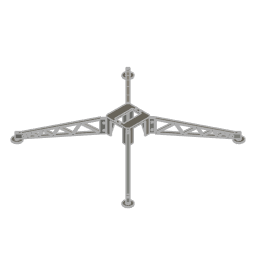
nerfaccelp3 v7 (Autodesk Fusion 360 design; units mm, degrees)
Autodesk Fusion 360 part; units mm, degrees
sketch "Sketch1" plane through (0, 0, 0) normal (0, 0, 1) x (1, 0, 0)
  line L0 (0, 0) -> (54, 0)
  line L1 (54, 0) -> (54, -54)
  line L2 (54, -54) -> (0, -54)
  line L3 (0, -54) -> (0, 0)
  line L4 (16.75, -6.5) -> (37.25, -6.5)
  line L5 (37.25, -6.5) -> (37.25, -47.5)
  line L6 (37.25, -47.5) -> (16.75, -47.5)
  line L7 (16.75, -47.5) -> (16.75, -6.5)
  line L8 (32, -2.725) -> (32, -51.275)
  line L9 (24.15, -2.725) -> (29.85, -2.725)
  line L10 (19.85, -2.725) -> (34.15, -2.725)
  circle A0 centre (32, -2.725) radius 2.15
  line L11 (22, -2.725) -> (32, -51.275)
  line L12 (37.25, -27) -> (16.75, -27)
  circle A1 centre (32, -2.725) radius 2
  line L13 (27, -27) -> (27, -2.725)
  circle A2 centre (22, -2.725) radius 2
  circle A3 centre (32, -51.275) radius 2
  circle A4 centre (22, -51.275) radius 2
  line L14 (54, 0) -> (0, -54)
  point P0 (27, -27)
  point P1 (32, -4.875)
  point P2 (32, -49.275)
  dimension "d1" = 20.5
  dimension "d2" = 41
  dimension "d4" = 5.7
  dimension "d5" = 14.3
  dimension "d6" = 4
  dimension "d7" = 44.4
  dimension "d8" = 54
  constraint horizontal L0
  constraint vertical L1
  constraint horizontal L2
  constraint vertical L3
  constraint coincident L0.start L3.end
  constraint horizontal L4
  constraint vertical L5
  constraint horizontal L6
  constraint vertical L7
  constraint perpendicular L6 L8
  constraint horizontal L9
  constraint horizontal L10
  constraint midpoint L9 L10
  constraint coincident L10 L8.start
  constraint coincident L10.end A0
  constraint coincident L9.end A0
  constraint coincident L8.start A0.centre
  constraint midpoint L5 L12.start
  constraint midpoint L7 L12.end
  constraint midpoint L12 P0
  constraint midpoint L11 P0
  constraint concentric A0 A1
  constraint coincident P0 L13.start
  constraint midpoint L9 L13.end
  constraint symmetric A1 L13 A2
  constraint symmetric L12 A1 A3
  constraint symmetric L12 A2 A4
  constraint coincident L10 L11.start
  constraint coincident L11.start A2.centre
  constraint midpoint P0 L14
  constraint equal L0 L1
  constraint coincident A0 P1
  constraint coincident L8 P1
  constraint coincident A3 P2
  constraint coincident L8 P2
  measures "d1" distance of L4.start L4.end
  measures "d2" distance of L4.end L5.end
  measures "d4" distance of L9.start L9.end
  measures "d5" distance of L10.start L10.end
  measures "d6" diameter of A1
  measures "d7" distance of P1 P2
  measures "d8" distance of L0.end L1.end
extrude "Extrude1" add sketch "Sketch1" along normal blind 4 contours L0 L3 L4 L5 L7 L8 L9 L10 A0 L11 A2 L14 | L1 L2 L5 L6 L7 L8 L11 A3 L14 | L4 L8 L9 L10 A0 L13 | L6 L8 L11 A3 | L4 L9 L10 L11 L13 A2 | L8 L10 A0 A1 | L8 L10 A0 A1 | L10 A0 A1 makes body 1
sketch "Sketch2" plane through (0, 0, 0) normal (0, 0, -1) x (1, 0, 0)
  circle A0 centre (22, 51.275) radius 2
  circle A1 centre (22, 2.725) radius 2
  circle A2 centre (32, 2.725) radius 2
  circle A3 centre (32, 51.275) radius 2
  line L0 (16.75, 47.5) -> (37.25, 47.5)
  line L1 (37.25, 47.5) -> (37.25, 6.5)
  line L2 (37.25, 6.5) -> (16.75, 6.5)
  line L3 (16.75, 6.5) -> (16.75, 47.5)
  line L4 (54, 54) -> (0, 54)
  line L5 (0, 54) -> (0, 0)
  line L6 (0, 0) -> (54, 0)
  line L7 (54, 0) -> (54, 54)
  line L8 (2, 49.8787) -> (2, 43.5147)
  line L9 (2, 43.5147) -> (10.4853, 52)
  line L10 (10.4853, 52) -> (4.1213, 52)
  line L11 (2, 49.8787) -> (4.1213, 52)
  line L12 (4.1213, 52) -> (4.1213, 54)
  line L13 (2, 49.8787) -> (0, 49.8787)
  line L14 (0, 38.6863) -> (15.3137, 54)
  line L15 (0, 38.6863) -> (19.9247, 38.6863) construction
  line L16 (27, 54) -> (27, 49.7302)
  line L17 (0, 27) -> (7.6569, 27)
  line L18 (43.5147, 52) -> (49.8787, 52)
  line L19 (52, 43.5147) -> (43.5147, 52)
  line L20 (52, 49.8787) -> (52, 43.5147)
  line L21 (52, 49.8787) -> (54, 49.8787)
  line L22 (49.8787, 52) -> (49.8787, 54)
  line L23 (54, 38.6863) -> (38.6863, 54)
  line L24 (52, 4.1213) -> (54, 4.1213)
  line L25 (52, 4.1213) -> (52, 10.4853)
  line L26 (52, 10.4853) -> (43.5147, 2)
  line L27 (43.5147, 2) -> (49.8787, 2)
  line L28 (49.8787, 2) -> (49.8787, 0)
  line L29 (54, 15.3137) -> (38.6863, 0)
  line L30 (0, 15.3137) -> (15.3137, 0)
  line L31 (2, 4.1213) -> (0, 4.1213)
  line L32 (2, 4.1213) -> (2, 10.4853)
  line L33 (2, 10.4853) -> (10.4853, 2)
  line L34 (10.4853, 2) -> (4.1213, 2)
  line L35 (4.1213, 2) -> (4.1213, 0)
  line L36 (6.5962, 45.2825) -> (12.253, 39.6256)
  line L37 (12.253, 39.6256) -> (14.3744, 41.747)
  line L38 (14.3744, 41.747) -> (8.7175, 47.4038)
  line L39 (6.5962, 45.2825) -> (8.7175, 47.4038)
  line L40 (47.4038, 45.2825) -> (45.2825, 47.4038)
  line L41 (47.4038, 45.2825) -> (41.747, 39.6256)
  line L42 (41.747, 39.6256) -> (39.6256, 41.747)
  line L43 (39.6256, 41.747) -> (45.2825, 47.4038)
  line L44 (47.4038, 8.7175) -> (45.2825, 6.5962)
  line L45 (47.4038, 8.7175) -> (41.747, 14.3744)
  line L46 (41.747, 14.3744) -> (39.6256, 12.253)
  line L47 (39.6256, 12.253) -> (45.2825, 6.5962)
  line L48 (6.5962, 8.7175) -> (8.7175, 6.5962)
  line L49 (6.5962, 8.7175) -> (12.253, 14.3744)
  line L50 (12.253, 14.3744) -> (14.3744, 12.253)
  line L51 (14.3744, 12.253) -> (8.7175, 6.5962)
  dimension "d11" = 45
  dimension "d12" = 12
  dimension "d13" = 3
  dimension "d14" = 2
  dimension "d15" = 2
  dimension "d16" = 45
  dimension "d17" = 2
  dimension "d18" = 3
  dimension "d19" = 8
  constraint perpendicular L4 L8
  constraint perpendicular L5 L10
  constraint coincident L8.start L11.start
  constraint parallel L9 L11
  constraint coincident L4 L12.end
  constraint perpendicular L4 L12
  constraint coincident L5 L13.end
  constraint perpendicular L5 L13
  constraint horizontal L15
  constraint coincident L5 L14.start
  constraint coincident L4 L14.end
  constraint midpoint L4 L16.start
  constraint perpendicular L4 L16
  constraint midpoint L5 L17.start
  constraint perpendicular L5 L17
  constraint symmetric L8.start L16 L20.start
  constraint symmetric L8.end L16 L19.start
  constraint symmetric L9.end L16 L18.start
  constraint symmetric L10.end L16 L18.end
  constraint symmetric L12.end L16 L22.end
  constraint symmetric L13.end L16 L21.end
  constraint symmetric L14.start L16 L23.start
  constraint symmetric L14.end L16 L23.end
  constraint symmetric L8.start L17 L31.start
  constraint symmetric L8.end L17 L32.end
  constraint symmetric L9.end L17 L33.end
  constraint symmetric L10.end L17 L34.end
  constraint symmetric L12.end L17 L35.end
  constraint symmetric L13.end L17 L31.end
  constraint symmetric L14.start L17 L30.start
  constraint symmetric L14.end L17 L30.end
  constraint symmetric L17 L18.start L26.end
  constraint symmetric L17 L18.end L27.end
  constraint symmetric L17 L19.start L25.end
  constraint symmetric L17 L20.start L24.start
  constraint symmetric L17 L21.end L24.end
  constraint symmetric L17 L22.end L28.end
  constraint symmetric L17 L23.start L29.start
  constraint symmetric L17 L23.end L29.end
  constraint coincident L14 L36.start
  constraint perpendicular L14 L36
  constraint perpendicular L36 L37
  constraint coincident L14 L38.end
  constraint perpendicular L14 L38
  constraint midpoint L14 L39
  constraint symmetric L16 L36.start L40.start
  constraint symmetric L16 L36.end L41.end
  constraint symmetric L16 L37.end L42.end
  constraint symmetric L16 L38.end L40.end
  constraint symmetric L17 L36.start L48.start
  constraint symmetric L17 L36.end L49.end
  constraint symmetric L17 L37.end L50.end
  constraint symmetric L17 L38.end L48.end
  constraint symmetric L17 L40.start L44.start
  constraint symmetric L17 L40.end L44.end
  constraint symmetric L17 L41.end L45.end
  constraint symmetric L17 L42.end L46.end
  measures "d11" angle of L8 L9
  measures "d12" distance of L8.end L9.end
  measures "d13" distance of L10.end L8.start
  measures "d14" distance of L10.end L12.end
  measures "d15" distance of L8.start L13.end
  measures "d16" angle of L14 L15
  measures "d17" distance of L9.end L14
  measures "d18" distance of L36.end L37.end
  measures "d19" distance of L36.start L36.end
extrude "Extrude2" add sketch "Sketch2" along normal blind 30 contours L4 L7 L18 L19 L20 L21 L22 L23 L40 | L23 L40 L41 L42 L43 | L6 L7 L24 L25 L26 L27 L28 L29 L44 | L4 L5 L8 L9 L10 L12 L13 L14 L39 | L29 L44 L45 L46 L47 | L14 L36 L37 L38 L39 | L5 L6 L30 L31 L32 L33 L34 L35 L48 | L30 L48 L49 L50 L51 bodies 1
chamfer "Chamfer1" distance 8 distance2 30 4 edges at (13.3137, -40.6863, -30) (40.6863, -40.6863, -30) (40.6863, -13.3137, -30) (13.3137, -13.3137, -30) measured on face at (11.0745, -42.2184, -30) measured on face at (42.9255, -42.2184, -30) measured on face at (42.9255, -11.7816, -30) measured on face at (11.7816, -11.0745, -30) on bodies 1
fillet "Fillet1" radius 0.5 8 edges at (2, -49.8787, -15) (4.1213, -52, -15) (52, -49.8787, -15) (49.8787, -52, -15) (49.8787, -2, -15) (52, -4.1213, -15) (2, -4.1213, -15) (4.1213, -2, -15) on bodies 1
sketch "Sketch3" plane through (0, 0, -30) normal (0, 0, -1) x (1, 0, 0)
  arc A0 (4.6213, 2) -> (4.1213, 1.5) centre (4.6213, 1.5) ccw
  line L0 (4.1213, 1.5) -> (4.1213, 0)
  line L1 (4.1213, 0) -> (15.3137, 0)
  line L2 (15.3137, 0) -> (8.7175, 6.5962)
  line L3 (6.5962, 8.7175) -> (0, 15.3137)
  line L4 (0, 15.3137) -> (0, 4.1213)
  line L5 (0, 4.1213) -> (1.5, 4.1213)
  arc A1 (1.5, 4.1213) -> (2, 4.6213) centre (1.5, 4.6213) ccw
  line L6 (2, 4.6213) -> (2, 10.4853)
  line L7 (2, 10.4853) -> (10.4853, 2)
  line L8 (10.4853, 2) -> (4.6213, 2)
  line L9 (1.4142, 13.8995) -> (0, 12.4853)
  line L10 (13.8995, 1.4142) -> (12.4853, 0)
  line L11 (8.7175, 6.5962) -> (6.5962, 8.7175)
  dimension "d26" = 2
  dimension "d27" = 2
  constraint coincident L3 L9.start
  constraint coincident L4 L9.end
  constraint perpendicular L3 L9
  constraint coincident L2 L10.start
  constraint coincident L1 L10.end
  constraint perpendicular L2 L10
  measures "d26" distance of L9.start L9.end
  measures "d27" distance of L10.start L10.end
extrude "Extrude3" cut sketch "Sketch3" against normal blind 30 contours L1 L2 L10 | L3 L4 L9 bodies 1
sketch "Sketch4" plane through (0, 0, -30) normal (0, 0, -1) x (1, 0, 0)
  arc A0 (4.1213, 52.5) -> (4.6213, 52) centre (4.6213, 52.5) ccw
  line L0 (4.6213, 52) -> (10.4853, 52)
  line L1 (10.4853, 52) -> (2, 43.5147)
  line L2 (2, 43.5147) -> (2, 49.3787)
  arc A1 (2, 49.3787) -> (1.5, 49.8787) centre (1.5, 49.3787) ccw
  line L3 (1.5, 49.8787) -> (0, 49.8787)
  line L4 (0, 49.8787) -> (0, 38.6863)
  line L5 (0, 38.6863) -> (6.5962, 45.2825)
  line L6 (8.7175, 47.4038) -> (15.3137, 54)
  line L7 (15.3137, 54) -> (4.1213, 54)
  line L8 (4.1213, 54) -> (4.1213, 52.5)
  line L9 (1.4142, 40.1005) -> (0, 41.5147)
  line L10 (13.8995, 52.5858) -> (12.4853, 54)
  line L11 (6.5962, 45.2825) -> (8.7175, 47.4038)
  dimension "d30" = 2
  dimension "d31" = 2
  constraint coincident L5 L9.start
  constraint coincident L4 L9.end
  constraint perpendicular L5 L9
  constraint coincident L6 L10.start
  constraint coincident L7 L10.end
  constraint perpendicular L6 L10
  measures "d30" distance of L10.start L10.end
  measures "d31" distance of L9.start L9.end
extrude "Extrude4" cut sketch "Sketch4" against normal blind 30 contours L6 L7 L10 | L4 L5 L9 bodies 1
sketch "Sketch5" plane through (0, 0, -30) normal (0, 0, -1) x (1, 0, 0)
  arc A0 (49.3787, 52) -> (49.8787, 52.5) centre (49.3787, 52.5) ccw
  line L0 (49.8787, 52.5) -> (49.8787, 54)
  line L1 (49.8787, 54) -> (38.6863, 54)
  line L2 (38.6863, 54) -> (45.2825, 47.4038)
  line L3 (47.4038, 45.2825) -> (54, 38.6863)
  line L4 (54, 38.6863) -> (54, 49.8787)
  line L5 (54, 49.8787) -> (52.5, 49.8787)
  arc A1 (52.5, 49.8787) -> (52, 49.3787) centre (52.5, 49.3787) ccw
  line L6 (52, 49.3787) -> (52, 43.5147)
  line L7 (52, 43.5147) -> (43.5147, 52)
  line L8 (43.5147, 52) -> (49.3787, 52)
  line L9 (40.2051, 52.4812) -> (41.7239, 54)
  line L10 (52.5858, 40.1005) -> (54, 41.5147)
  line L11 (45.2825, 47.4038) -> (47.4038, 45.2825)
  dimension "d36" = 2.1479
  dimension "d45" = 2
  constraint coincident L2 L9.start
  constraint coincident L1 L9.end
  constraint perpendicular L2 L9
  constraint coincident L3 L10.start
  constraint coincident L4 L10.end
  constraint perpendicular L3 L10
  measures "d36" distance of L9.start L9.end
  measures "d45" distance of L10.start L10.end
extrude "Extrude5" cut sketch "Sketch5" against normal blind 30 contours L1 L2 L9 | L3 L4 L10 bodies 1
sketch "Sketch6" plane through (0, 0, -30) normal (0, 0, -1) x (1, 0, 0)
  arc A0 (52, 4.6213) -> (52.5, 4.1213) centre (52.5, 4.6213) ccw
  line L0 (52.5, 4.1213) -> (54, 4.1213)
  line L1 (54, 4.1213) -> (54, 15.3137)
  line L2 (54, 15.3137) -> (47.4038, 8.7175)
  line L3 (45.2825, 6.5962) -> (38.6863, 0)
  line L4 (38.6863, 0) -> (49.8787, 0)
  line L5 (49.8787, 0) -> (49.8787, 1.5)
  arc A1 (49.8787, 1.5) -> (49.3787, 2) centre (49.3787, 1.5) ccw
  line L6 (49.3787, 2) -> (43.5147, 2)
  line L7 (43.5147, 2) -> (52, 10.4853)
  line L8 (52, 10.4853) -> (52, 4.6213)
  line L9 (52.5858, 13.8995) -> (54, 12.4853)
  line L10 (40.1005, 1.4142) -> (41.5147, 0)
  line L11 (47.4038, 8.7175) -> (45.2825, 6.5962)
  dimension "d40" = 2
  dimension "d44" = 2
  constraint coincident L2 L9.start
  constraint coincident L1 L9.end
  constraint perpendicular L2 L9
  constraint coincident L3 L10.start
  constraint coincident L4 L10.end
  constraint perpendicular L3 L10
  measures "d40" distance of L9.start L9.end
  measures "d44" distance of L10.start L10.end
extrude "Extrude6" cut sketch "Sketch6" against normal blind 30 contours L1 L2 L9 | L3 L4 L10 bodies 1
chamfer "Chamfer2" distance 4 angle 45 4 edges at (0, 0, 2) (54, 0, 2) (54, -54, 2) (0, -54, 2) on bodies 1
chamfer "Chamfer3" distance 2 angle 45 16 edges at (49.9948, -11.3085, 0) (44.5754, -11.5459, 0) (42.6915, -4.0052, 0) (42.4541, -9.4246, 0) (49.9948, -42.6915, 0) (42.7438, -49.9425, 0) (42.4541, -44.5754, 0) (44.5754, -42.4541, 0) (4.0052, -42.6915, 0) (9.4246, -42.4541, 0) (11.5459, -44.5754, 0) (11.3085, -49.9948, 0) (11.5459, -9.4246, 0) (11.3085, -4.0052, 0) (9.4246, -11.5459, 0) (4.0052, -11.3085, 0) on bodies 1
sketch "Sketch7" plane through (0, 0, -30) normal (0, 0, -1) x (1, 0, 0)
  line L0 (12.4853, 0) -> (13.8995, 1.4142)
  line L1 (13.8995, 1.4142) -> (8.7175, 6.5962)
  line L2 (6.5962, 8.7175) -> (1.4142, 13.8995)
  line L3 (1.4142, 13.8995) -> (0, 12.4853)
  line L4 (0, 12.4853) -> (0, 4.1213)
  line L5 (0, 4.1213) -> (1.5, 4.1213)
  arc A0 (1.5, 4.1213) -> (2, 4.6213) centre (1.5, 4.6213) ccw
  line L6 (2, 4.6213) -> (2, 10.4853)
  line L7 (2, 10.4853) -> (10.4853, 2)
  line L8 (10.4853, 2) -> (4.6213, 2)
  arc A1 (4.6213, 2) -> (4.1213, 1.5) centre (4.6213, 1.5) ccw
  line L9 (4.1213, 1.5) -> (4.1213, 0)
  line L10 (4.1213, 0) -> (12.4853, 0)
  line L11 (9.761, 2.3) -> (2.3, 9.761)
  line L12 (2.3, 9.761) -> (2.3, 4.0678)
  line L13 (9.761, 2.3) -> (4.0678, 2.3)
  line L14 (4.0678, 2.3) -> (2.3, 4.0678)
  line L15 (4.0678, 2.3) -> (2.6536, 0.8858)
  line L16 (2.3, 4.0678) -> (0.8858, 2.6536)
  line L17 (3.891, -0.3517) -> (-0.3517, 3.891)
  line L18 (2.6536, 0.8858) -> (0.8858, 2.6536)
  line L19 (3.891, -0.3517) -> (-102.175, -106.4177)
  line L20 (-102.175, -106.4177) -> (-106.4177, -102.175)
  line L21 (-106.4177, -102.175) -> (-0.3517, 3.891)
  line L22 (8.7175, 6.5962) -> (6.5962, 8.7175)
  line L23 (2.6536, 0.8858) -> (-3.0033, -4.7711)
  line L24 (-3.0033, -4.7711) -> (-4.7711, -3.0033)
  line L25 (-4.7711, -3.0033) -> (0.8858, 2.6536)
  dimension "d48" = 0.3
  dimension "d49" = 0.3
  dimension "d50" = 0.3
  dimension "d51" = 2.5
  dimension "d52" = 2
  dimension "d53" = 150
  dimension "d54" = 6
  dimension "d65" = 8
  constraint parallel L7 L11
  constraint perpendicular L8 L12
  constraint parallel L8 L13
  constraint parallel L11 L14
  constraint perpendicular L14 L15
  constraint perpendicular L14 L16
  constraint equal L15 L16
  constraint coincident L16.end L17
  constraint coincident L15.end L17
  constraint midpoint L17 L18
  constraint perpendicular L17 L19
  constraint perpendicular L19 L20
  constraint parallel L19 L21
  constraint parallel L15 L23
  constraint perpendicular L23 L24
  constraint perpendicular L24 L25
  measures "d48" distance of L8 L13
  measures "d49" distance of L7 L11
  measures "d50" distance of L6 L12
  measures "d51" distance of L12.end L13.end
  measures "d52" distance of L13.end L15.end
  measures "d53" distance of L17.start L19.end
  measures "d54" distance of L17.start L17.end
  measures "d65" distance of L15.end L23.end
extrude "Extrude20" add sketch "Sketch7" against normal blind 30 separate body contours L11 L12 L13 L14 | L14 L15 L16 L17 L18 | L17 L18 L23 L24 L25 makes body 2
sketch "Sketch16" plane through (-0.8839, -0.8839, 0) normal (-0.707107, -0.707107, 0) x (0.707107, -0.707107, 0)
  line L0 (-5.4973, -30) -> (4.5027, -30)
  line L1 (4.5027, -30) -> (4.5027, 0)
  line L2 (4.5027, 0) -> (-5.4973, 0)
  line L3 (-5.4973, 0) -> (-5.4973, -30)
  line L4 (1.5027, 0) -> (1.5027, -30)
  line L5 (-5.4973, 0) -> (-138.4973, -30)
  line L6 (-138.4973, -30) -> (-148.4973, -30)
  line L7 (-148.4973, -30) -> (-148.4973, -40)
  line L8 (-148.4973, -40) -> (-138.4973, -40)
  line L9 (-138.4973, -40) -> (-5.4973, -30)
  line L10 (-138.4973, -30) -> (-138.4973, -40)
  dimension "d111" = 7
  dimension "d112" = 10
  dimension "d113" = 10
  dimension "d115" = 10
  dimension "d123" = 150
  constraint coincident L2 L4.start
  constraint coincident L0 L4.end
  constraint perpendicular L0 L4
  constraint coincident L2.end L3.start
  constraint perpendicular L3 L6
  constraint perpendicular L6 L7
  constraint perpendicular L7 L8
  constraint coincident L0.start L3.end
  constraint vertical L10
  measures "d111" distance of L2.end L4.start
  measures "d112" distance of L6.end L7.end
  measures "d113" distance of L5.end L6.end
  measures "d115" vertical distance of L8.end L0.start
  measures "d123" horizontal distance of L4.end L7.end
extrude "Extrude21" add sketch "Sketch16" along normal blind 2 separate body contours L0 L2 L3 L4 | L3 L5 L9 L10 | L6 L7 L8 L10 makes body 3
sketch "Sketch17" plane through (-0.8839, -0.8839, 0) normal (0.707107, 0.707107, 0) x (-0.707107, 0.707107, 0)
  line L0 (5.4973, 0) -> (-1.5027, 0)
  line L1 (-1.5027, 0) -> (-1.5027, -30)
  line L2 (-1.5027, -30) -> (5.4973, -30)
  line L3 (5.4973, -30) -> (138.4973, -40)
  line L4 (138.4973, -40) -> (148.4973, -40)
  line L5 (148.4973, -40) -> (148.4973, -30)
  line L6 (148.4973, -30) -> (138.4973, -30)
  line L7 (138.4973, -30) -> (5.4973, 0)
  line L8 (5.4973, 0) -> (5.4973, -30)
  constraint coincident L0.start L7.end
  constraint coincident L2.end L3.start
extrude "Extrude22" add sketch "Sketch17" along normal blind 4.5 separate body contours L3 L4 L5 L6 L7 L8 makes body 4
combine "Combine2" operation add target body 3 tool bodies 4
extrude "Extrude24" cut 1 faces at (-1.4712, -0.2965, -20) along direction (-0.707107, -0.707107, 0) blind 0.5 on bodies 3 bodies 3
sketch "Sketch18" plane through (0.8839, 0.8839, 0) normal (0.707107, 0.707107, 0) x (-0.707107, 0.707107, 0)
  line L0 (-4.5027, -30) -> (5.4973, -30)
  line L1 (5.4973, -30) -> (5.4973, 0)
  line L2 (5.4973, 0) -> (-4.5027, 0)
  line L3 (-4.5027, 0) -> (-4.5027, -30)
  circle A0 centre (1.4973, -8) radius 2
  circle A1 centre (1.4973, -23) radius 2
  line L4 (1.4973, -8) -> (1.4973, -23)
  dimension "d128" = 4
  dimension "d129" = 4
  dimension "d130" = 15
  dimension "d131" = 7
  dimension "d133" = 4
  constraint coincident A0.centre L4.start
  constraint coincident A1.centre L4.end
  constraint vertical L4
  measures "d128" diameter of A0
  measures "d129" diameter of A1
  measures "d130" vertical distance of A0.centre A1.centre
  measures "d131" vertical distance of L0.end A1.centre
  measures "d133" horizontal distance of L1.end A0.centre
extrude "Extrude25" cut sketch "Sketch18" against normal blind 4.5 contours A0 | A1 bodies 2 3
sketch "Sketch20" plane through (0, 0, -40) normal (0, 0, -1) x (1, 0, 0)
  line L0 (-95.6343, -100.2305) -> (-100.2305, -95.6343)
  line L1 (-100.2305, -95.6343) -> (-107.3016, -102.7054)
  line L2 (-107.3016, -102.7054) -> (-102.7054, -107.3016)
  line L3 (-102.7054, -107.3016) -> (-95.6343, -100.2305)
  line L4 (-102.7054, -107.3016) -> (-102.7054, -98.1092)
  line L5 (-102.7054, -98.1092) -> (-107.3016, -102.7054)
  circle A0 centre (-102.7054, -102.7054) radius 2
  dimension "d136" = 4
  constraint coincident L2.end L3.start
  constraint coincident L1 L4.end
  constraint coincident L1.end L2.start
  constraint perpendicular L2 L5
  constraint equal L2 L5
  constraint midpoint L4 A0.centre
  measures "d136" diameter of A0
extrude "Extrude26" cut sketch "Sketch20" against normal blind 10 contours L4 A0 | L4 A0 bodies 3
sketch "Sketch22" plane through (2.2981, 2.2981, 0) normal (0.707107, 0.707107, 0) x (-0.707107, 0.707107, 0)
  line L0 (5.4973, 0) -> (5.4973, -30)
  line L1 (5.4973, -30) -> (138.4973, -40)
  line L2 (138.4973, -40) -> (148.4973, -40)
  line L3 (148.4973, -40) -> (148.4973, -30)
  line L4 (148.4973, -30) -> (138.4973, -30)
  line L5 (138.4973, -30) -> (5.4973, 0)
  line L6 (6.4973, -0.2256) -> (6.4973, -30.0752)
  dimension "d139" = 1
  constraint coincident L5 L6.start
  constraint coincident L1 L6.end
  constraint parallel L0 L6
  measures "d139" horizontal distance of L0.end L6.end
extrude "Extrude27" cut sketch "Sketch22" against normal blind 5 contours L0 L1 L5 L6 bodies 3
sketch "Sketch23" plane through (2.2981, 2.2981, 0) normal (0.707107, 0.707107, 0) x (-0.707107, 0.707107, 0)
  line L0 (6.4973, -0.2256) -> (6.4973, -30.0752)
  line L1 (6.4973, -30.0752) -> (138.4973, -40)
  line L2 (138.4973, -40) -> (148.4973, -40)
  line L3 (148.4973, -40) -> (148.4973, -30)
  line L4 (148.4973, -30) -> (138.4973, -30)
  line L5 (138.4973, -30) -> (6.4973, -0.2256)
  line L6 (138.4973, -30) -> (138.4973, -40)
  line L7 (136.4973, -31.5991) -> (8.4973, -2.7269)
  line L8 (8.4973, -2.7269) -> (8.4973, -28.2199)
  line L9 (8.4973, -28.2199) -> (136.4973, -37.844)
  line L10 (136.4973, -31.5991) -> (136.4973, -37.844)
  line L11 (8.4973, -28.2199) -> (39.6296, -9.7493)
  line L12 (39.6296, -9.7493) -> (52.5535, -31.5324)
  line L13 (52.5535, -31.5324) -> (75.5952, -17.8618)
  line L14 (75.5952, -17.8618) -> (85.1605, -33.9841)
  line L15 (85.1605, -33.9841) -> (102.2143, -23.8661)
  line L16 (102.2143, -23.8661) -> (109.2938, -35.7986)
  line L17 (109.2938, -35.7986) -> (121.9158, -28.3101)
  line L18 (121.9158, -28.3101) -> (127.1555, -37.1416)
  line L19 (127.1555, -37.1416) -> (136.4973, -31.5991)
  line L20 (9.0076, -29.0799) -> (39.2798, -11.1195)
  line L21 (39.2798, -11.1195) -> (52.2037, -32.9027)
  line L22 (52.2037, -32.9027) -> (75.2455, -19.2321)
  line L23 (75.2455, -19.2321) -> (84.8107, -35.3543)
  line L24 (84.8107, -35.3543) -> (101.8645, -25.2364)
  line L25 (101.8645, -25.2364) -> (108.944, -37.1689)
  line L26 (108.944, -37.1689) -> (121.566, -29.6803)
  line L27 (121.566, -29.6803) -> (126.8057, -38.5119)
  line L28 (126.8057, -38.5119) -> (137.0076, -32.4591)
  line L29 (7.9871, -27.3599) -> (39.9794, -8.379)
  line L30 (39.9794, -8.379) -> (52.9032, -30.1621)
  line L31 (52.9032, -30.1621) -> (75.945, -16.4915)
  line L32 (75.945, -16.4915) -> (85.5103, -32.6138)
  line L33 (85.5103, -32.6138) -> (102.5641, -22.4958)
  line L34 (102.5641, -22.4958) -> (109.6436, -34.4283)
  line L35 (109.6436, -34.4283) -> (122.2655, -26.9398)
  line L36 (122.2655, -26.9398) -> (127.5053, -35.7713)
  line L37 (127.5053, -35.7713) -> (135.9871, -30.7391)
  dimension "d142" = -2
  dimension "d143" = 1
  dimension "d144" = -1
  constraint coincident L4.end L5.start
  constraint coincident L1.end L2.start
  constraint coincident L7 L11.end
  constraint coincident L9 L12.end
  constraint perpendicular L11 L12
  constraint coincident L7 L13.end
  constraint perpendicular L12 L13
  constraint coincident L9 L14.end
  constraint perpendicular L13 L14
  constraint coincident L7 L15.end
  constraint perpendicular L14 L15
  constraint coincident L9 L16.end
  constraint perpendicular L15 L16
  constraint coincident L7 L17.end
  constraint perpendicular L16 L17
  constraint coincident L9 L18.end
  constraint perpendicular L17 L18
  constraint perpendicular L18 L19
extrude "Extrude28" cut sketch "Sketch23" against normal blind 6.5 contours L7 L36 L37 | L9 L10 L28 | L9 L26 L27 | L7 L34 L35 | L9 L24 L25 | L7 L32 L33 | L9 L22 L23 | L7 L30 L31 | L9 L20 L21 | L7 L8 L29 bodies 3
sketch "Sketch24" plane through (0, 0, -40) normal (0, 0, -1) x (1, 0, 0)
  circle A0 centre (-102.7054, -102.7054) radius 2
  line L0 (-95.6343, -100.2305) -> (-100.2305, -95.6343)
  line L1 (-100.2305, -95.6343) -> (-107.3016, -102.7054)
  line L2 (-107.3016, -102.7054) -> (-102.7054, -107.3016)
  line L3 (-102.7054, -107.3016) -> (-95.6343, -100.2305)
  circle A1 centre (-102.7054, -102.7054) radius 4
  dimension "d147" = 8
  constraint concentric A0 A1
  measures "d147" diameter of A1
extrude "Extrude29" add sketch "Sketch24" along normal blind 2 separate body contours A0 | L3 A1 | L1 L2 L3 A1 | L1 A1 | L2 A1 makes body 5
sketch "Sketch25" plane through (0, 0, -42) normal (0, 0, -1) x (1, 0, 0)
  circle A0 centre (-102.7054, -102.7054) radius 4
  circle A1 centre (-102.7054, -102.7054) radius 3
  dimension "d150" = 1
  constraint concentric A0 A1
  measures "d150" distance of A0 A1
extrude "Extrude30" add sketch "Sketch25" along normal blind 3 bodies 5
sketch "Sketch26" plane through (0, 0, -45) normal (0, 0, -1) x (1, 0, 0)
  circle A0 centre (-102.7054, -102.7054) radius 3
  circle A1 centre (-102.7054, -102.7054) radius 4
  circle A2 centre (-102.7054, -102.7054) radius 10
  dimension "d153" = 20
  constraint concentric A0 A2
  measures "d153" diameter of A2
extrude "Extrude31" add sketch "Sketch26" against normal blind 2 separate body contours A2 makes body 6
combine "Combine3" operation add target body 5 tool bodies 6
extrude "Extrude32" cut sketch "Sketch24" along normal blind 2 contours A0 bodies 5
ref_plane "WorkPlane2" through (27, -27, -13) normal (0, 1, 0) x (-1, 0, 0)
sketch "Sketch27" plane through (0, -27, 0) normal (0, 1, 0) x (1, 0, 0)
  line L0 (0, -4) -> (54, -4)
  line L1 (27, -4) -> (27, -13.9835)
  point P0 (54, -4)
  point P1 (0, -4)
  constraint horizontal L0
  constraint coincident P0 L0.end
  constraint coincident L0.start P1
  constraint midpoint L0 L1.start
  constraint perpendicular L0 L1
pattern_circular "C-Pattern4" count 4 over 360 about axis through (27, -27, 4) along (0, 0, 1) of bodies 2 3 5 makes body 7 at (4.787, -46.726, -20) makes body 8 at (46.726, -49.213, -20) makes body 9 at (49.213, -7.274, -10) makes body 10 at (-100.3483, -158.9445, -33.3333) makes body 11 at (158.9445, -154.3483, -33.3333) makes body 12 at (151.9913, 102.5875, -36.6667) makes body 13 at (-103.2022, -149.0759, -45) makes body 14 at (160.0898, -163.561, -45) makes body 15 at (160.5927, 96.1218, -45)
equation "d20 = h"
equation "d23 = h"
equation "d28 = -h"
equation "d32 = -h"
equation "d37 = -h"
equation "d42 = -h"
equation "h = 30 mm"
equation "d118 = 2.50 mm + 2 mm"
equation "d158 = -54.00 mm / 2"
